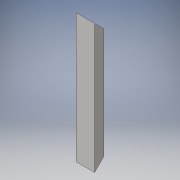
# Autodesk Inventor part: graber back peice
Saved by Autodesk Inventor 2016 SP2 (Build 200236200, 236)
## iProperties
Created: 2018-01-19
Part Number: graber back peice
Material: Generic
Document SubType Name: Modeling
Designer: CAD
Density: 1 g/cm^3
Appearance: Default
Author: CAD
Autodesk Inventor part; units mm, degrees
ref_plane "YZ Plane" through (0, 0, 0) normal (1, 0, 0) x (0, 1, 0)
ref_plane "XZ Plane" through (0, 0, 0) normal (0, 1, 0) x (-1, 0, 0)
ref_plane "XY Plane" through (0, 0, 0) normal (0, 0, 1) x (1, 0, 0)
sketch "Sketch1" plane through (0, 0, 0) normal (0, 1, 0) x (-1, 0, 0)
  line L0 (0, 0) -> (50.8, 0)
  line L1 (50.8, 0) -> (50.8, -25.4)
  line L2 (50.8, -25.4) -> (0, -25.4)
  line L3 (0, -25.4) -> (0, 0)
  dimension "d0" = 50.8
  dimension "d1" = 25.4
  constraints: 8 end point, 2 parallel, 1 horizontal, 1 perpendicular
  measures "d0" distance of L1.end L2.end
  measures "d1" distance of L0.end L1.end
extrude "Extrusion1" add sketch "Sketch1" along normal blind 355.6
sketch "Sketch3" plane through (0, 0, 0) normal (1, 0, 0) x (0, 0, -1)
  line L0 (25.4, 0) -> (0, 0) projected
  line L1 (25.4, 0) -> (25.4, 25.4)
  line L2 (25.4, 0) -> (25.4, 355.6) projected
  line L3 (0, 0) -> (0, 355.6) projected
  line L4 (25.4, 25.4) -> (0, 0)
  line L5 (0, 177.8) -> (104.5089, 177.8)
  line L6 (0, 0) -> (25.4, 0)
  line L7 (25.4, 355.6) -> (0, 355.6)
  line L8 (25.4, 355.6) -> (25.4, 330.2)
  line L9 (25.4, 330.2) -> (0, 355.6)
  line L10 (0, 355.6) -> (25.4, 355.6)
  dimension "d4" = 25.4
  constraints: 16 end point, 1 collinear, 1 horizontal, 1 midpoint, 1 point on line, 1 symmetric about line
  measures "d4" distance of L0.start L1.end
shell "Shell1" thickness 1.905 removed faces 2 at (-16.9333, 0, -16.9333) at (-16.9333, 355.6, -16.9333)
extrude "Extrusion2" cut sketch "Sketch3" against normal blind 355.6 contours L0 L4 L1 | L7 L2 L9
body "Solid1"
